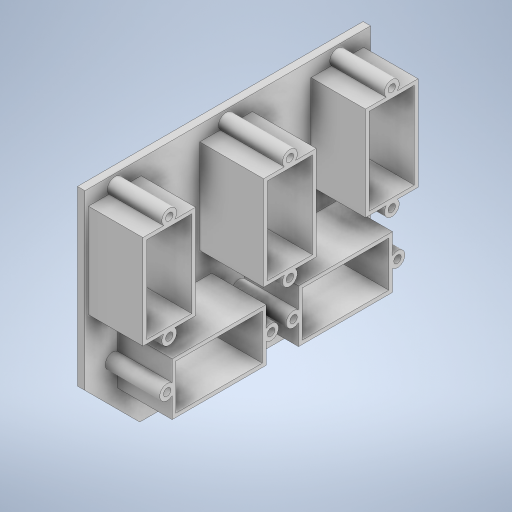
# Autodesk Inventor part: Palm_ServoAttachment
Saved by Autodesk Inventor 2023 (Build 270158000, 158)
## iProperties
Created: 2023-04-20
Part Number: Palm_ServoAttachment
Material: Generic
Document SubType Name: Modeling
Designer: 1senadi
Density: 1 g/cm^3
Appearance: Default
Author: 1senadi
Autodesk Inventor part; units mm, degrees
ref_plane "YZ Plane" through (0, 0, 0) normal (1, 0, 0) x (0, 1, 0)
ref_plane "XZ Plane" through (0, 0, 0) normal (0, 1, 0) x (-1, 0, 0)
ref_plane "XY Plane" through (0, 0, 0) normal (0, 0, 1) x (1, 0, 0)
sketch "Sketch1" plane through (0, 0, 0) normal (1, 0, 0) x (0, 1, 0)
  line L0 (0, 0) -> (0, -76)
  line L1 (0, 0) -> (76, 0) construction
  line L2 (0, -76) -> (-46, -76)
  line L3 (-46, -76) -> (-46, 0)
  line L4 (-46, 0) -> (0, 0)
  dimension "d0" = 76
  dimension "d1" = 90
  dimension "d2" = 46
  constraints: 10 end point, 3 perpendicular, 2 horizontal, 1 vertical
  measures "d0" distance of L0.start L0.end
  measures "d1" angle of L0 L1
  measures "d2" distance of L0.end L2.end
extrude "Extrusion1" add sketch "Sketch1" along normal blind 2
sketch "Sketch2" plane through (0, 0, 0) normal (-1, 0, 0) x (0, 0, 1)
  line L0 (-76, -46) -> (-76, 0) projected
  line L1 (-76, 0) -> (-73.12, 0)
  line L2 (-76, 0) -> (0, 0) projected
  line L3 (-73.12, 0) -> (-73.12, -5)
  line L4 (-73.12, -5) -> (-61.12, -5)
  line L5 (-61.12, -5) -> (-61.12, -28)
  line L6 (-61.12, -28) -> (-73.12, -28)
  line L7 (-73.12, -28) -> (-73.12, -5)
  line L8 (-73.12, -5) -> (-37.52, -5)
  line L9 (-37.52, -5) -> (-1.92, -5)
  line L10 (-1.92, -5) -> (-1.92, -28)
  line L11 (-1.92, -28) -> (-13.92, -28)
  line L12 (-13.92, -28) -> (-13.92, -5)
  line L13 (-37.52, -5) -> (-31.52, -5)
  line L14 (-31.52, -5) -> (-31.52, -28)
  line L15 (-31.52, -28) -> (-43.52, -28)
  line L16 (-43.52, -28) -> (-43.52, -5)
  line L17 (-67.12, -28) -> (-67.12, -30.313)
  line L18 (-67.12, -5) -> (-67.12, -2.687)
  circle A0 centre (-67.12, -2.687) radius 1
  circle A1 centre (-67.12, -30.313) radius 1
  line L19 (-37.52, -28) -> (-37.52, -30.313)
  line L20 (-37.52, -5) -> (-37.52, -2.687)
  line L21 (-7.92, -5) -> (-7.92, -2.687)
  line L22 (-7.92, -28) -> (-7.92, -30.313)
  circle A2 centre (-37.52, -2.687) radius 1
  circle A3 centre (-7.92, -2.687) radius 1
  circle A4 centre (-37.52, -30.313) radius 1
  circle A5 centre (-7.92, -30.313) radius 1
  dimension "d5" = 2.88
  dimension "d6" = 5
  dimension "d7" = 12
  dimension "d8" = 23
  dimension "d9" = 12
  dimension "d10" = 35.6
  dimension "d14" = 35.6
  dimension "d15" = 23
  dimension "d16" = 12
  dimension "d17" = 6
  dimension "d18" = 23
  dimension "d19" = 12
  dimension "d24" = 2.313
  dimension "d25" = 2.313
  dimension "d26" = 2
  dimension "d27" = 2
  dimension "d28" = 2
  dimension "d29" = 2
  dimension "d30" = 2
  dimension "d31" = 2
  constraints: 42 end point, 9 perpendicular, 6 centre point, 6 coincident, 6 point on line, 6 vertical, 3 horizontal, 3 midpoint
  measures "d5" distance of L0.end L1.end
  measures "d6" distance of L1.end L3.end
  measures "d7" distance of L3.end L4.end
  measures "d8" distance of L4.end L5.end
  measures "d9" distance of L5.end L6.end
  measures "d10" distance of L3.end L8.end
  measures "d14" distance of L8.end L9.end
  measures "d15" distance of L9.end L10.end
  measures "d16" distance of L10.end L11.end
  measures "d17" distance of L8.end L13.end
  measures "d18" distance of L13.end L14.end
  measures "d19" distance of L14.end L15.end
  measures "d24" distance of L17.start L17.end
  measures "d25" distance of L18.start L18.end
  measures "d26" diameter of A0
  measures "d27" diameter of A1
  measures "d28" diameter of A2
  measures "d29" diameter of A3
  measures "d30" diameter of A4
  measures "d31" diameter of A5
extrude "Extrusion2" cut sketch "Sketch2" against normal up to surface (2 mm away)
sketch "Sketch11" plane through (2, 0, 0) normal (1, 0, 0) x (0, 0, -1)
  line L0 (0, -46) -> (76, -46) projected
  line L1 (0, -46) -> (14.5664, -60.5664)
  line L2 (0, -46) -> (20.6, -46) construction
  line L3 (76, -46) -> (61.4336, -60.5664)
  line L4 (76, -46) -> (96.6, -46) construction
  line L5 (61.4336, -60.5664) -> (14.5664, -60.5664)
  point P0 (0, 0)
  dimension "d94" = 20.6
  dimension "d95" = 45
  dimension "d96" = 20.6
  dimension "d97" = 135
  constraints: 10 end point, 2 equal length, 2 horizontal
  measures "d94" distance of L0.start L1.end
  measures "d95" angle of L1 L2
  measures "d96" distance of L0.end L3.end
  measures "d97" angle of L3 L4
extrude "Extrusion9" add sketch "Sketch11" against normal up to surface (2 mm away)
sketch "Sketch14" plane through (2, 0, 0) normal (1, 0, 0) x (0, 0, -1)
  line L0 (1.92, -5) -> (13.92, -5) projected
  line L1 (1.92, -28) -> (1.92, -5) projected
  line L2 (13.92, -28) -> (1.92, -28) projected
  circle A0 centre (7.92, -30.313) radius 1 projected
  line L3 (13.92, -5) -> (13.92, -28) projected
  circle A1 centre (7.92, -2.687) radius 1 projected
  line L4 (14.92, -29) -> (0.92, -29)
  line L5 (0.92, -29) -> (0.92, -4)
  line L6 (0.92, -4) -> (14.92, -4)
  line L7 (14.92, -4) -> (14.92, -29)
  circle A2 centre (7.92, -2.687) radius 2
  circle A3 centre (7.92, -30.313) radius 2
  point P0 (0, 0)
  point P1 (9.4287, -4)
  point P2 (6.4113, -4)
  point P3 (6.4113, -29)
  point P4 (9.4287, -29)
  dimension "d112" = 1
  dimension "d113" = 1
  dimension "d114" = 1
  constraints: 8 end point, 2 centre point, 3 other
  measures "d112" distance between parallel lines of L3 L7
  measures "d113" radial gap between concentric circles of A1 A2
  measures "d114" radial gap between concentric circles of A0 A3
extrude "Extrusion12" add sketch "Sketch14" along normal blind 14.5
sketch "Sketch15" plane through (2, 0, 0) normal (1, 0, 0) x (0, 0, -1)
  line L0 (31.52, -5) -> (43.52, -5) projected
  line L1 (43.52, -5) -> (43.52, -28) projected
  line L2 (31.52, -28) -> (31.52, -5) projected
  line L3 (43.52, -28) -> (31.52, -28) projected
  circle A0 centre (37.52, -30.313) radius 1 projected
  circle A1 centre (37.52, -2.687) radius 1 projected
  line L4 (44.52, -29) -> (44.52, -4)
  line L5 (44.52, -4) -> (30.52, -4)
  line L6 (30.52, -4) -> (30.52, -29)
  line L7 (30.52, -29) -> (44.52, -29)
  circle A2 centre (37.52, -2.687) radius 2
  circle A3 centre (37.52, -30.313) radius 2
  point P0 (0, 0)
  point P1 (39.0287, -4)
  point P2 (36.0113, -4)
  point P3 (36.0113, -29)
  point P4 (39.0287, -29)
  dimension "d117" = 1
  dimension "d118" = 1
  dimension "d119" = 1
  constraints: 8 end point, 2 centre point, 3 other
  measures "d117" distance between parallel lines of L1 L4
  measures "d118" radial gap between concentric circles of A1 A2
  measures "d119" radial gap between concentric circles of A0 A3
extrude "Extrusion13" add sketch "Sketch15" along normal blind 17
sketch "Sketch16" plane through (2, 0, 0) normal (1, 0, 0) x (0, 0, -1)
  line L0 (61.12, -5) -> (73.12, -5) projected
  line L1 (73.12, -5) -> (73.12, -28) projected
  line L2 (61.12, -28) -> (61.12, -5) projected
  line L3 (73.12, -28) -> (61.12, -28) projected
  circle A0 centre (67.12, -30.313) radius 1 projected
  circle A1 centre (67.12, -2.687) radius 1 projected
  line L4 (74.12, -4) -> (60.12, -4)
  line L5 (60.12, -4) -> (60.12, -29)
  line L6 (60.12, -29) -> (74.12, -29)
  line L7 (74.12, -29) -> (74.12, -4)
  circle A2 centre (67.12, -2.687) radius 2
  circle A3 centre (67.12, -30.313) radius 2
  point P0 (0, 0)
  point P1 (65.6113, -29)
  point P2 (68.6287, -29)
  point P3 (68.6287, -4)
  point P4 (65.6113, -4)
  dimension "d134" = 90
  dimension "d136" = 0
  dimension "d122" = 1
  dimension "d123" = 1
  dimension "d124" = 1
  constraints: 8 end point, 2 centre point, 3 other
  measures "d122" distance between parallel lines of L0 L4
  measures "d123" radial gap between concentric circles of A1 A2
  measures "d124" radial gap between concentric circles of A0 A3
extrude "Extrusion14" add sketch "Sketch16" along normal blind 14.5
sketch "Sketch17" plane through (2, 0, 0) normal (1, 0, 0) x (0, 0, -1)
  line L0 (76, 0) -> (0, 0) projected
  line L1 (38, 0) -> (38, -60.5664)
  line L2 (14.5664, -60.5664) -> (61.4336, -60.5664) projected
  line L3 (38, -42.813) -> (35, -42.813)
  circle A0 centre (35, -42.813) radius 1
  arc A1 (33.687, -44.3217) -> (33.687, -41.3043) centre (35, -42.813) ccw
  line L4 (35, -42.813) -> (32.687, -42.813)
  line L5 (32.687, -42.813) -> (32.687, -36.813)
  line L6 (32.687, -36.813) -> (9.687, -36.813)
  line L7 (9.687, -36.813) -> (9.687, -48.813)
  line L8 (9.687, -48.813) -> (32.687, -48.813)
  line L9 (9.687, -48.813) -> (32.687, -48.813) construction
  line L10 (32.687, -48.813) -> (32.687, -42.813)
  line L11 (9.687, -42.813) -> (7.374, -42.813)
  circle A2 centre (7.374, -42.813) radius 1
  arc A3 (8.687, -41.3043) -> (8.687, -44.3217) centre (7.374, -42.813) ccw
  line L12 (8.687, -35.813) -> (33.687, -35.813)
  line L13 (33.687, -35.813) -> (33.687, -42.813)
  line L14 (33.687, -42.813) -> (33.687, -49.813)
  line L15 (33.687, -49.813) -> (8.687, -49.813)
  line L16 (8.687, -49.813) -> (8.687, -35.813)
  circle A4 centre (41, -42.813) radius 1
  arc A5 (42.313, -41.3043) -> (42.313, -44.3217) centre (41, -42.813) ccw
  line L17 (43.313, -42.813) -> (43.313, -36.813)
  line L18 (43.313, -36.813) -> (66.313, -36.813)
  line L19 (66.313, -36.813) -> (66.313, -48.813)
  line L20 (66.313, -48.813) -> (43.313, -48.813)
  line L21 (43.313, -48.813) -> (43.313, -42.813)
  circle A6 centre (68.626, -42.813) radius 1
  arc A7 (67.313, -44.3217) -> (67.313, -41.3043) centre (68.626, -42.813) ccw
  line L22 (67.313, -35.813) -> (42.313, -35.813)
  line L23 (42.313, -35.813) -> (42.313, -42.813)
  line L24 (42.313, -42.813) -> (42.313, -49.813)
  line L25 (42.313, -49.813) -> (67.313, -49.813)
  line L26 (67.313, -49.813) -> (67.313, -35.813)
  dimension "d127" = 3
  dimension "d128" = 2
  dimension "d129" = 1
  dimension "d130" = 2.313
  dimension "d131" = 6
  dimension "d132" = 23
  dimension "d133" = 12
  dimension "d134" = 90
  dimension "d135" = 23
  dimension "d136" = 0
  dimension "d137" = 2.313
  dimension "d138" = 2
  dimension "d139" = 1
  dimension "d140" = 1
  constraints: 50 end point, 16 symmetric about line, 9 point on line, 8 centre point, 8 point on circle, 6 perpendicular, 4 horizontal, 2 coincident, 2 midpoint, 1 collinear, 8 other
  measures "d127" distance of L3.start L3.end
  measures "d128" diameter of A0
  measures "d129" radial gap between concentric circles of A0 A1
  measures "d130" distance of L4.start L4.end
  measures "d131" distance of L4.end L5.end
  measures "d132" distance of L5.end L6.end
  measures "d133" distance of L6.end L7.end
  measures "d134" angle of L7 L6
  measures "d135" distance of L7.end L8.end
  measures "d136" distance between parallel lines of L8 L9
  measures "d137" distance of L11.start L11.end
  measures "d138" diameter of A2
  measures "d139" radial gap between concentric circles of A2 A3
  measures "d140" distance between parallel lines of L6 L12
extrude "Extrusion15" add sketch "Sketch17" along normal blind 14.5 contours A0 L4 L13 A1 L3 | L3 A1 L14 L4 A0 | L14 L15 L16 L11 L7 L8 L10 L4 | L13 L4 L5 L6 L7 L11 L16 L12 | A3 L16 | L23 L24 A5 | L23 L22 L26 L25 L24 | A7 L26
sketch "Sketch18" plane through (2, 0, 0) normal (1, 0, 0) x (0, 0, -1)
  line L0 (9.687, -48.813) -> (32.687, -48.813) projected
  line L1 (32.687, -48.813) -> (32.687, -36.813) projected
  line L2 (32.687, -36.813) -> (9.687, -36.813) projected
  line L3 (9.687, -36.813) -> (9.687, -48.813) projected
  line L4 (43.313, -36.813) -> (43.313, -48.813) projected
  line L5 (43.313, -48.813) -> (66.313, -48.813) projected
  line L6 (66.313, -48.813) -> (66.313, -36.813) projected
  line L7 (66.313, -36.813) -> (43.313, -36.813) projected
  circle A0 centre (35, -42.813) radius 1 projected
  circle A1 centre (7.374, -42.813) radius 1 projected
  circle A2 centre (41, -42.813) radius 1 projected
  circle A3 centre (68.626, -42.813) radius 1 projected
  point P0 (0, 0)
extrude "Extrusion16" cut sketch "Sketch18" against normal up to surface (2 mm away)
body "Solid1"
